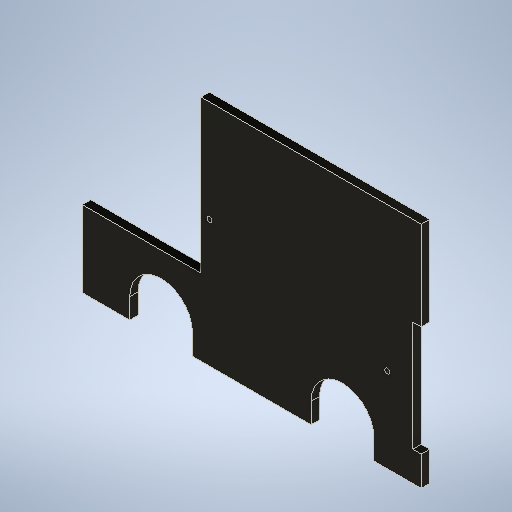
# Autodesk Inventor part: SIDE_1
Saved by Autodesk Inventor 2025.3 (Build 293356030, 356C)
## iProperties
Created: 2026-06-30
Part Number: SIDE_1
Material: ABS Plastic
Document SubType Name: Modeling
Designer: user
Density: 1.06 g/cm^3
Appearance: Gunmetal
Author: user
Autodesk Inventor part; units mm, degrees
ref_plane "YZ Plane" through (0, 0, 0) normal (1, 0, 0) x (0, 1, 0)
ref_plane "XZ Plane" through (0, 0, 0) normal (0, 1, 0) x (-1, 0, 0)
ref_plane "XY Plane" through (0, 0, 0) normal (0, 0, 1) x (1, 0, 0)
sketch "Sketch1" plane through (0, 0, 0) normal (0, 0, 1) x (1, 0, 0)
  line L0 (200, 0) -> (200, 135)
  line L1 (200, 135) -> (70, 135)
  line L2 (0, 45) -> (0, 0)
  line L3 (70, 45) -> (0, 45)
  line L4 (0, 45) -> (0, 0)
  line L5 (70, 45) -> (70, 135)
  line L6 (0, 0) -> (28, 0)
  line L7 (0, 0) -> (28, 0)
  line L8 (0, 0) -> (28, 0)
  line L9 (54, 0) -> (70, 0)
  line L10 (70, 0) -> (70, 135) construction
  arc A0 (172, 12) -> (135, 12) centre (153.5, 12) ccw
  line L11 (135, 0) -> (135, 12)
  line L12 (172, 0) -> (172, 12)
  arc A1 (65, 12) -> (28, 12) centre (46.5, 12) ccw
  line L13 (28, 0) -> (28, 12)
  line L14 (65, 0) -> (65, 12)
  line L15 (54, 0) -> (135, 0)
  line L16 (200, 17.5) -> (195, 17.5)
  line L17 (195, 17.5) -> (195, 82.5)
  line L18 (195, 82.5) -> (200, 82.5)
  line L19 (200, 82.5) -> (200, 17.5)
  line L20 (172, 0) -> (200, 0)
  point P0 (200, 82.5)
  dimension "d14" = 200
  dimension "d15" = 70
  dimension "d17" = 37
  dimension "d19" = 37
  dimension "d23" = 5
  dimension "d24" = 65
  dimension "d27" = 28
  dimension "d28" = 52.5
  dimension "d47" = 45
  dimension "d48" = 135
  dimension "d49" = 28
  constraints: 42 end point, 9 parallel, 6 horizontal, 4 point on circle, 3 perpendicular, 3 vertical, 2 centre point, 2 point on line
  measures "d14" distance between parallel lines of L2 L0
  measures "d15" distance of L3.start L2.start
  measures "d17" distance between parallel lines of L12 L11
  measures "d19" distance between parallel lines of L14 L13
  measures "d23" distance of L17.end L18.end
  measures "d24" distance of L16.end L17.end
  measures "d27" distance of L12.start L0.start
  measures "d28" distance between parallel lines of L18 L1
  measures "d47" distance of L2.start L2.end
  measures "d48" distance of L0.start L0.end
  measures "d49" distance between parallel lines of L2 L13
extrude "Extrusion1" add sketch "Sketch1" along normal blind 5 contours L20 L12 A0 L11 L15 L9 L14 A1 L13 L6 L2 L3 L5 L1 L0 L18 L17 L16
sketch "Sketch2" plane through (0, 0, 5) normal (0, 0, 1) x (1, 0, 0)
  line L0 (195, 17.5) -> (195, 82.5) projected
  line L1 (200, 17.5) -> (195, 17.5) projected
  point P0 (0, 0)
  point P1 (180, 50)
  dimension "d36" = 15
  dimension "d37" = 32.5
  measures "d36" distance from line of L0 point (180, 50)
  measures "d37" distance from line of L1 point (180, 50)
hole "Hole1" at (180, 50, 5) direction (0, 0, -1) diameter 3 end through all
sketch "Sketch3" plane through (0, 0, 5) normal (0, 0, 1) x (1, 0, 0)
  line L0 (70, 135) -> (70, 45) projected
  line L1 (70, 45) -> (0, 45) projected
  point P0 (0, 0)
  point P1 (75, 75)
  dimension "d45" = 5
  dimension "d46" = 30
  measures "d45" distance from line of L0 point (75, 75)
  measures "d46" distance from line of point (75, 75) L1
hole "Hole2" at (75, 75, 5) direction (0, 0, -1) diameter 3 end through all
body "Solid1"
